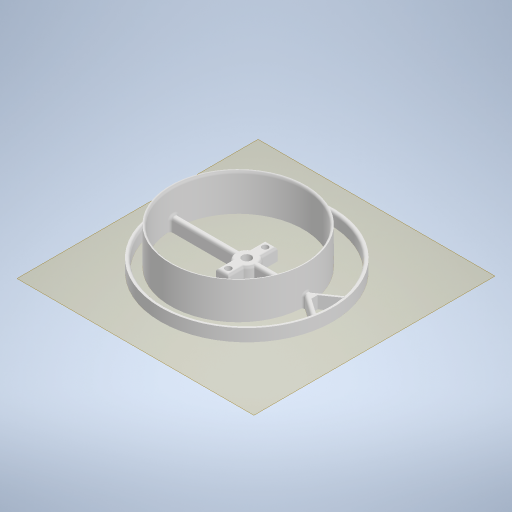
# Autodesk Inventor part: SkimmerLidInsert
Saved by Autodesk Inventor 2023.2 (Build 272271030, 271C)
## iProperties
Created: 2023-02-16
Part Number: SkimmerLidInsert
Material: Generic
Document SubType Name: Modeling
Designer: atrus
Density: 1 g/cm^3
Appearance: Default
Author: atrus
Autodesk Inventor part; units mm, degrees
ref_plane "YZ Plane" through (0, 0, 0) normal (1, 0, 0) x (0, 1, 0)
ref_plane "XZ Plane" through (0, 0, 0) normal (0, 1, 0) x (-1, 0, 0)
ref_plane "XY Plane" through (0, 0, 0) normal (0, 0, 1) x (1, 0, 0)
sketch "Sketch1" plane through (0, 0, 0) normal (0, 1, 0) x (-1, 0, 0)
  circle A0 centre (0, 0) radius 70
  circle A1 centre (0, 0) radius 3.675
  line L0 (66.9533, 2.5) -> (8.6458, 2.5)
  line L1 (8.6458, -2.5) -> (66.9533, -2.5)
  line L2 (8.6458, 2.5) -> (8.6458, -2.5) construction
  line L3 (-8.6458, -2.5) -> (-49.7621, -2.5)
  line L4 (-55, -2.5) -> (-55, 2.5)
  line L5 (-49.7621, 2.5) -> (-8.6458, 2.5)
  line L6 (-55, -2.5) -> (-66.1996, -10.3251)
  line L7 (-49.7621, -2.5) -> (-65.6107, -13.5734)
  line L8 (-49.7621, 2.5) -> (-65.6107, 13.5734)
  line L9 (-55, 2.5) -> (-66.1996, 10.3251)
  arc A2 (66.9533, 2.5) -> (-65.6107, 13.5734) centre (0, 0) ccw
  arc A3 (-66.1996, 10.3251) -> (-66.1996, -10.3251) centre (0, 0) ccw
  arc A4 (-65.6107, -13.5734) -> (66.9533, -2.5) centre (0, 0) ccw
  line L10 (0, 0) -> (-55, 0) construction
  line L11 (-8.6458, -2.5) -> (-8.6458, 2.5) construction
  line L12 (5, -20) -> (-5, -20)
  line L13 (-5, -20) -> (-5, -7.4833)
  line L14 (5, -7.4833) -> (5, -20)
  line L15 (-5, 7.4833) -> (-5, 20)
  line L16 (-5, 20) -> (5, 20)
  line L17 (5, 20) -> (5, 7.4833)
  circle A5 centre (0, -15) radius 2.5 projected
  circle A6 centre (0, 15) radius 2.5 projected
  line L18 (0, -20) -> (0, 20) construction
  arc A7 (8.6458, 2.5) -> (5, 7.4833) centre (0, 0) ccw
  arc A8 (-5, 7.4833) -> (-8.6458, 2.5) centre (0, 0) ccw
  arc A9 (-8.6458, -2.5) -> (-5, -7.4833) centre (0, 0) ccw
  arc A10 (5, -7.4833) -> (8.6458, -2.5) centre (0, 0) ccw
  point P0 (8.6458, 0)
  dimension "d1" = 140
  dimension "d2" = 7.35
  dimension "d4" = 5
  dimension "d12" = 3
  dimension "d14" = 3
  dimension "d15" = 3
  dimension "d16" = 55
  dimension "d17" = 5
  dimension "d18" = 10
  dimension "d19" = 10
  dimension "d20" = 12.5167
  dimension "d21" = 49.8248
  constraints: 38 end point, 14 point on circle, 9 centre point, 6 parallel, 5 equal length, 5 perpendicular, 4 coincident, 4 horizontal, 4 midpoint, 3 concentric, 2 point on line, 1 collinear, 1 horizontal alignment
  measures "d1" diameter of A0
  measures "d2" diameter of A1
  measures "d4" distance between parallel lines of L1 L0
  measures "d12" distance between parallel lines of L6 L7
  measures "d14" radial gap between concentric circles of A0 A4
  measures "d15" radial gap between concentric circles of A0 A3
  measures "d16" distance of L10.start L10.end
  measures "d17" distance from line of L12 A5.centre
  measures "d18" distance of L12.start L12.end
  measures "d19" distance of L13.end L14.start
  measures "d20" distance of L12.end L13.end
  measures "d21" distance of L10.start L3.end
extrude "Extrusion1" add sketch "Sketch1" along normal blind 10
fillet "Fillet2" radius 2 19 edges at (29.2039, 10, 2.5) (29.2039, 10, -2.5) (-37.7996, 10, -2.5) (-37.7996, 10, 2.5) (57.6864, 10, -8.0367) (57.6864, 10, 8.0367) (67, 10, 0) (-5.5772, 10, -66.7675) (-5.5772, 10, 66.7675) (-5, 10, -13.7417) (5, 10, -13.7417) (0, 10, -20) (-5, 10, 13.7417) (5, 10, 13.7417) (0, 10, 20) (-7.2636, 10, 5.3141) (-7.2636, 10, -5.3141) (7.2636, 10, -5.3141) (7.2636, 10, 5.3141)
ref_plane "Work Plane1" through (7.5, 0, 0) normal (0, 1, 0) x (1, 0, 0)
sketch "Sketch2" plane through (7.5, 0, 0) normal (0, 1, 0) x (1, 0, 0)
  line L0 (-7.5, 0) -> (-144.819, 0) construction
  line L1 (-14.4821, -0.5) -> (-76.4982, -0.5) construction
  circle A0 centre (-14.5, 0) radius 55
  circle A1 centre (-14.5, 0) radius 53
  dimension "d23" = 110
  dimension "d24" = 7
  dimension "d25" = 2
  constraints: 2 centre point, 2 end point, 1 coincident, 1 parallel, 1 point on line
  measures "d23" diameter of A0
  measures "d24" distance of L0.start A0.centre
  measures "d25" radial gap between concentric circles of A0 A1
extrude "Extrusion2" add sketch "Sketch2" along normal blind 30
fillet "Fillet3" radius 2 1 edges at (-60, 30, 0)
fillet "Fillet4" radius 2 16 edges at (45.9994, 10, 0.25) (45.9994, 10, -0.25) (45.9616, 9.3041, -2.0163) (45.941, 4, -2.5) (45.941, 4, 2.5) (45.9615, 9.3016, 2.0185) (-59.9616, 9.3041, 2.0163) (-59.941, 4, 2.5) (-59.9616, 9.3041, -2.0163) (-59.941, 4, -2.5) (-60, 10, 0) (-62, 10, 0) (-61.963, 9.3041, -2.0163) (-61.9432, 4, -2.5) (-61.9432, 4, 2.5) (-61.963, 9.3041, 2.0163)
fillet "Fillet5" radius 1.5 6 edges at (47.9629, 9.3016, 2.0185) (47.9432, 4, 2.5) (47.963, 9.3041, -2.0163) (47.9432, 4, -2.5) (47.9994, 10, -0.25) (47.9994, 10, 0.25)
body "Solid1"
